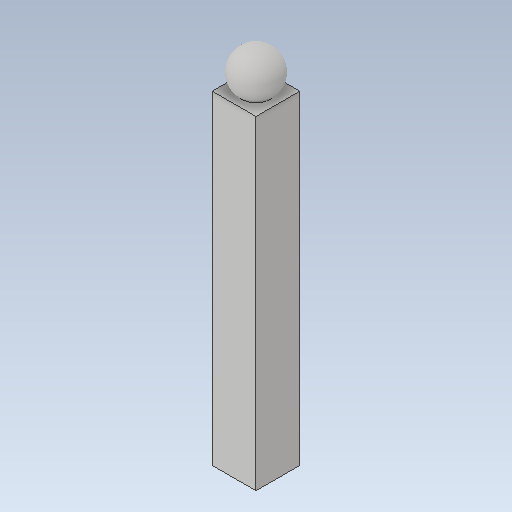
# Autodesk Inventor part: Central Part
Saved by Autodesk Inventor 2021 (Build 250183000, 183)
## iProperties
Created: 2020-12-28
Part Number: Central Part
Material: Generic
Document SubType Name: Modeling
Designer: Thomas Dodd
Density: 1 g/cm^3
Appearance: Default
Author: Thomas Dodd
Autodesk Inventor part; units mm, degrees
ref_plane "YZ Plane" through (0, 0, 0) normal (1, 0, 0) x (0, 1, 0)
ref_plane "XZ Plane" through (0, 0, 0) normal (0, 1, 0) x (-1, 0, 0)
ref_plane "XY Plane" through (0, 0, 0) normal (0, 0, 1) x (1, 0, 0)
sketch "Sketch1" plane through (0, 0, 0) normal (0, 1, 0) x (-1, 0, 0)
  line L0 (0, 0) -> (40, 0)
  line L1 (40, 0) -> (40, -40)
  line L2 (40, -40) -> (0, -40)
  line L3 (0, -40) -> (0, 0)
  dimension "d0" = 40
  dimension "d1" = 40
  constraints: 8 end point, 2 parallel, 1 horizontal, 1 perpendicular
  measures "d0" distance of L1.end L2.end
  measures "d1" distance of L0.end L1.end
extrude "Extrusion1" add sketch "Sketch1" along normal blind 296
sketch "Sketch3" plane through (0, 296, 0) normal (0, 1, 0) x (1, 0, 0)
  line L0 (-40, 0) -> (0, 0) projected
  line L1 (0, 0) -> (0, 40) projected
  line L2 (0, 40) -> (-40, 40) projected
  line L3 (-40, 40) -> (-40, 0) projected
extrude "Extrusion3" add sketch "Sketch3" along normal blind 40 separate body
ref_plane "Work Plane1" through (-20, 296, 0) normal (1, 0, 0) x (0, 0, -1)
sketch "Sketch4" plane through (-20, 296, 0) normal (1, 0, 0) x (0, 0, -1)
  arc A0 (20, 35.3125) -> (7.1343, 0) centre (20, 15.3125) ccw
  line L0 (20, 35.3125) -> (20, 47.82)
  line L1 (20, 47.82) -> (-11.6226, 47.82)
  line L2 (-11.6226, 47.82) -> (-11.6226, 0)
  line L3 (-11.6226, 0) -> (0, 0)
  line L4 (-11.6226, 0) -> (7.1343, 0)
  point P0 (0, -296)
  constraints: 10 end point, 2 perpendicular, 2 point on circle, 2 vertical, 1 centre point, 1 coincident
revolve "Revolution1" cut sketch "Sketch4" angle 360 about axis through (-20, 331.3125, -20) along (0, 1, 0) bodies 2
sketch "Sketch5" plane through (0, 0, 0) normal (1, 0, 0) x (0, 0, -1)
  line L0 (40, 0) -> (0, 0) projected
  line L1 (40, 0) -> (40, 296) projected
  line L2 (0, 296) -> (40, 296) projected
  line L3 (0, 0) -> (0, 296) projected
  line L4 (7.1343, 296) -> (32.8657, 296) projected
  arc A0 (32.8657, 296) -> (7.1343, 296) centre (20, 311.3125) ccw projected
body "Solid1"
body "Solid2"
